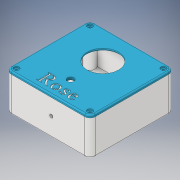
# Autodesk Inventor part: Box
Saved by Autodesk Inventor 2018.3 (Build 223284000, 284)
## iProperties
Created: 2018-06-03
Part Number: Box
Material: Generisch
Document SubType Name: Modeling
Designer: JochenAlt
Density: 1 g/cm^3
Appearance: Vorgabe
Author: JochenAlt
Autodesk Inventor part; units mm, degrees
ref_plane "YZ Plane" through (0, 0, 0) normal (1, 0, 0) x (0, 1, 0)
ref_plane "XZ Plane" through (0, 0, 0) normal (0, 1, 0) x (-1, 0, 0)
ref_plane "XY Plane" through (0, 0, 0) normal (0, 0, 1) x (1, 0, 0)
sketch "Skizze1" plane through (0, 0, 0) normal (0, 0, 1) x (1, 0, 0)
  line L0 (57, -65) -> (-57, -65)
  line L1 (-65, -57) -> (-65, 57)
  line L2 (-57, 65) -> (57, 65)
  line L3 (65, 57) -> (65, -57)
  line L4 (65, -65) -> (-65, 65) construction
  line L5 (-65, -65) -> (65, 65) construction
  arc A0 (65, 57) -> (57, 65) centre (57, 57) ccw
  line L6 (-57, 57) -> (57, 57) construction
  line L7 (57, 57) -> (57, -57) construction
  line L8 (57, -57) -> (-57, -57) construction
  line L9 (-57, -57) -> (-57, 57) construction
  circle A1 centre (-57, 57) radius 1.5
  circle A2 centre (57, 57) radius 1.5
  circle A3 centre (-57, -57) radius 1.5
  circle A4 centre (57, -57) radius 1.5
  circle A5 centre (-57, 57) radius 4
  circle A6 centre (57, 57) radius 4
  circle A7 centre (-57, -57) radius 4
  circle A8 centre (57, -57) radius 4
  line L10 (50.755, 62) -> (-50.755, 62)
  line L11 (-62, 50.755) -> (-62, -50.755)
  line L12 (-50.755, -62) -> (50.755, -62)
  line L13 (62, -50.755) -> (62, 50.755)
  arc A9 (-65, -57) -> (-57, -65) centre (-57, -57) ccw
  arc A10 (-50.755, -62) -> (-62, -50.755) centre (-57, -57) ccw
  arc A11 (62, -50.755) -> (50.755, -62) centre (57, -57) ccw
  arc A12 (50.755, 62) -> (62, 50.755) centre (57, 57) ccw
  arc A13 (-57, 65) -> (-65, 57) centre (-57, 57) ccw
  arc A14 (-62, 50.755) -> (-50.755, 62) centre (-57, 57) ccw
  line L14 (-62, 50.755) -> (-62, 62) construction
  line L15 (-50.755, 62) -> (-62, 62) construction
  line L16 (50.755, 62) -> (62, 62) construction
  line L17 (62, 50.755) -> (62, 62) construction
  line L18 (-62, -50.755) -> (-62, -62) construction
  line L19 (-50.755, -62) -> (-62, -62) construction
  line L20 (50.755, -62) -> (62, -62) construction
  line L21 (62, -50.755) -> (62, -62) construction
  line L22 (-55.1236, 60.25) -> (-53.2472, 57)
  line L23 (-53.2472, 57) -> (-55.1236, 53.75)
  line L24 (-55.1236, 53.75) -> (-58.8764, 53.75)
  line L25 (-58.8764, 53.75) -> (-60.7528, 57)
  line L26 (-60.7528, 57) -> (-58.8764, 60.25)
  line L27 (-58.8764, 60.25) -> (-55.1236, 60.25)
  line L28 (58.8764, 60.25) -> (60.7528, 57)
  line L29 (60.7528, 57) -> (58.8764, 53.75)
  line L30 (58.8764, 53.75) -> (55.1236, 53.75)
  line L31 (55.1236, 53.75) -> (53.2472, 57)
  line L32 (53.2472, 57) -> (55.1236, 60.25)
  line L33 (55.1236, 60.25) -> (58.8764, 60.25)
  line L34 (55.1236, -53.75) -> (58.8764, -53.75)
  line L35 (58.8764, -53.75) -> (60.7528, -57)
  line L36 (60.7528, -57) -> (58.8764, -60.25)
  line L37 (58.8764, -60.25) -> (55.1236, -60.25)
  line L38 (55.1236, -60.25) -> (53.2472, -57)
  line L39 (53.2472, -57) -> (55.1236, -53.75)
  line L40 (-53.2472, -57) -> (-55.1236, -60.25)
  line L41 (-55.1236, -60.25) -> (-58.8764, -60.25)
  line L42 (-58.8764, -60.25) -> (-60.7528, -57)
  line L43 (-60.7528, -57) -> (-58.8764, -53.75)
  line L44 (-58.8764, -53.75) -> (-55.1236, -53.75)
  line L45 (-55.1236, -53.75) -> (-53.2472, -57)
  arc A15 (57, -65) -> (65, -57) centre (57, -57) ccw
  point P0 (0, 0)
  dimension "d0" = 130
  dimension "d1" = 130
  dimension "d3" = 3
  dimension "d4" = 8
  dimension "d11" = 8
  dimension "d12" = 3
  dimension "d54" = 6.5
  constraints: 92 end point, 16 centre point, 16 point on circle, 15 point on line, 14 coincident, 12 equal radius, 11 perpendicular, 6 parallel, 6 tangent, 5 equal length, 4 horizontal, 2 midpoint, 2 vertical, 1 collinear, 52 other
  measures "d0" distance of L4.end L5.end
  measures "d1" distance of L5.end L4.start
  measures "d3" diameter of A1
  measures "d4" diameter of A5
  measures "d11" radius of A13
  measures "d12" distance between parallel lines of L10 L2
  measures "d54" distance between parallel lines of L24 L27
extrude "Extrusion1" add sketch "Skizze1" along normal blind 2 contours L0 A9 L1 A13 L2 A0 L3 A15 | A12 L13 A11 L12 A10 L11 A14 L10
extrude "Extrusion2" add sketch "Skizze1" along normal blind 2 from surface at 2 contours L0 A9 L1 A13 L2 A0 L3 A15 | A5 | A6 | A7 | A8 | A12 L13 A11 L12 A10 L11 A14 L10 | L22 L23 L24 L25 L26 L27 | L28 L29 L30 L31 L32 L33 | L34 L35 L36 L37 L38 L39 | L40 L41 L42 L43 L44 L45
extrude "Extrusion3" add sketch "Skizze1" along normal blind 50 from surface at 4 contours L0 A9 L1 A13 L2 A0 L3 A15 | A5 | A6 | A7 | A8 | L22 L23 L24 L25 L26 L27 | L28 L29 L30 L31 L32 L33 | L34 L35 L36 L37 L38 L39 | L40 L41 L42 L43 L44 L45
extrude "Extrusion4" add sketch "Skizze1" along normal blind 2 from surface at 54 separate body contours L0 A9 L1 A13 L2 A0 L3 A15 | A5 | A6 | A7 | A8 | A12 L13 A11 L12 A10 L11 A14 L10 | L22 L23 L24 L25 L26 L27 | L28 L29 L30 L31 L32 L33 | L34 L35 L36 L37 L38 L39 | L40 L41 L42 L43 L44 L45
extrude "Extrusion5" add sketch "Skizze1" along normal blind 2 from surface at 56 contours L0 A9 L1 A13 L2 A0 L3 A15 | A12 L13 A11 L12 A10 L11 A14 L10 bodies 2
extrude "Extrusion9" cut sketch "Skizze1" against normal blind 12 from surface at 54 contours L22 L23 L24 L25 L26 L27 | L28 L29 L30 L31 L32 L33 | L34 L35 L36 L37 L38 L39 | L40 L41 L42 L43 L44 L45 bodies 1
fillet "Rundung1" radius 2 7 edges at (65, 0, 0) (62.6569, 62.6569, 0) (0, 65, 0) (-62.6569, 62.6569, 0) (-65, 0, 0) (-62.6569, -62.6569, 0) (0, -65, 0)
fillet "Rundung2" radius 2 7 edges at (-62.6569, -62.6569, 58) (-65, 0, 58) (-62.6569, 62.6569, 58) (0, 65, 58) (62.6569, 62.6569, 58) (65, 0, 58) (0, -65, 58)
sketch "Skizze2" plane through (-57, 63, 58) normal (0, 0, 1) x (1, 0, 0)
  circle A0 centre (57, -43) radius 24.25
  circle A1 centre (57, -43) radius 25.5
  circle A2 centre (57, -93) radius 5
  circle A3 centre (57, -43) radius 28.5
  circle A4 centre (57, -43) radius 29
  point P0 (57, -63)
  dimension "d22" = 48.5
  dimension "d28" = 51
  dimension "d29" = 20
  dimension "d30" = 10
  dimension "d31" = 50
  dimension "d63" = 3
  dimension "d68" = 0.5
  constraints: 5 centre point, 3 coincident
  measures "d22" diameter of A0
  measures "d28" diameter of A1
  measures "d29" distance of A0.centre point (57, -63)
  measures "d30" diameter of A2
  measures "d31" distance of A2.centre A0.centre
  measures "d63" radial gap between concentric circles of A3 A1
  measures "d68" radial gap between concentric circles of A4 A3
extrude "Extrusion6" cut sketch "Skizze2" against normal up to next contours A0 | A2 bodies 2
extrude "Extrusion7" cut sketch "Skizze2" along normal blind 2 from surface at -4 contours A1 bodies 2
sketch "Odroid" plane through (0, 0, 0) normal (0, 0, 1) x (1, 0, 0)
  line L0 (-51, 9.5) -> (7, 9.5) construction
  line L1 (7, 9.5) -> (7, -39.5) construction
  line L2 (7, -39.5) -> (-51, -39.5) construction
  line L3 (-51, -39.5) -> (-51, 9.5) construction
  circle A0 centre (-51, 9.5) radius 1.4
  circle A1 centre (7, 9.5) radius 1.4
  circle A2 centre (7, -39.5) radius 1.4
  circle A3 centre (-51, -39.5) radius 1.4
  line L4 (-52.5, 13) -> (28.5, 13)
  line L5 (30.5, 11) -> (30.5, -41)
  line L6 (28.5, -43) -> (-52.5, -43)
  line L7 (-54.5, -41) -> (-54.5, 11)
  line L8 (-54.5, 13) -> (30.5, -43) construction
  line L9 (-54.5, -43) -> (30.5, 13) construction
  line L10 (-51, -15) -> (7, -15) construction
  arc A4 (-52.5, 13) -> (-54.5, 11) centre (-52.5, 11) ccw
  arc A5 (30.5, 11) -> (28.5, 13) centre (28.5, 11) ccw
  arc A6 (28.5, -43) -> (30.5, -41) centre (28.5, -41) ccw
  arc A7 (-54.5, -41) -> (-52.5, -43) centre (-52.5, -41) ccw
  circle A8 centre (-51, -39.5) radius 2.5
  circle A9 centre (7, -39.5) radius 2.5
  circle A10 centre (7, 9.5) radius 2.5
  circle A11 centre (-51, 9.5) radius 2.5
  line L11 (-54.5, 42) -> (-0.5, 42)
  line L12 (-0.5, 42) -> (-0.5, 18)
  line L13 (-0.5, 18) -> (-54.5, 18)
  line L14 (-54.5, 18) -> (-54.5, 42)
  circle A12 centre (-45.7, 39.5) radius 2.5
  circle A13 centre (-9.3, 20.5) radius 2.5
  circle A14 centre (-9.3, 20.5) radius 1.4
  circle A15 centre (-45.7, 39.5) radius 1.4
  line L15 (0.5, 42) -> (54.5, 42)
  line L16 (54.5, 42) -> (54.5, 18)
  line L17 (54.5, 18) -> (0.5, 18)
  line L18 (0.5, 18) -> (0.5, 42)
  circle A16 centre (9.3, 39.5) radius 2.5
  circle A17 centre (45.7, 20.5) radius 2.5
  circle A18 centre (45.7, 20.5) radius 1.4
  circle A19 centre (9.3, 39.5) radius 1.4
  line L19 (50.755, 62) -> (-50.755, 62) construction
  arc A20 (-62, 50.755) -> (-50.755, 62) centre (-57, 57) ccw construction
  line L20 (-62, 50.755) -> (-62, -50.755) construction
  arc A21 (-50.755, -62) -> (-62, -50.755) centre (-57, -57) ccw construction
  line L21 (-50.755, -62) -> (50.755, -62) construction
  arc A22 (62, -50.755) -> (50.755, -62) centre (57, -57) ccw construction
  line L22 (62, -50.755) -> (62, 50.755) construction
  arc A23 (50.755, 62) -> (62, 50.755) centre (57, 57) ccw construction
  line L23 (0, 91) -> (0, -91) construction
  line L24 (-91, 0) -> (91, 0) construction
  point P0 (0, 0)
  point P1 (-12, -15)
  point P2 (-12, -15)
  dimension "d32" = 58
  dimension "d33" = 49
  dimension "d34" = 2.8
  dimension "d35" = 56
  dimension "d36" = 85
  dimension "d37" = 3.5
  dimension "d38" = 15
  dimension "d39" = 12
  dimension "d40" = 2
  dimension "d41" = 5
  dimension "d47" = 24
  dimension "d49" = 2.5
  dimension "d50" = 2.5
  dimension "d51" = 8.8
  dimension "d53" = 8.8
  dimension "d73" = 24
  dimension "d74" = 2.5
  dimension "d75" = 2.5
  dimension "d76" = 8.8
  dimension "d77" = 8.8
  dimension "d78" = 1
  dimension "d87" = 54
  dimension "d88" = 20
  constraints: 38 end point, 20 centre point, 15 equal radius, 12 coincident, 9 point on line, 8 parallel, 8 point on circle, 8 tangent, 4 horizontal, 4 midpoint, 4 perpendicular, 2 collinear, 1 other
  measures "d32" distance of L0.start L0.end
  measures "d33" distance of L0.end L1.end
  measures "d34" diameter of A0
  measures "d35" distance of L9.end L8.end
  measures "d36" distance of L8.start L9.end
  measures "d37" distance between parallel lines of L3 L7
  measures "d38" vertical distance of point (-12, -15) point (0, 0)
  measures "d39" horizontal distance of point (-12, -15) point (0, 0)
  measures "d40" radius of A4
  measures "d41" diameter of A8
  measures "d47" distance of L11.end L12.end
  measures "d49" distance from line of L11 A12.centre
  measures "d50" distance from line of L13 A13.centre
  measures "d51" distance from line of A12.centre L14
  measures "d53" distance from line of L12 A13.centre
  measures "d73" distance of L16.start L16.end
  measures "d74" distance from line of L15 A16.centre
  measures "d75" distance from line of L17 A17.centre
  measures "d76" distance from line of A16.centre L18
  measures "d77" distance from line of L16 A17.centre
  measures "d78" distance between parallel lines of L18 L12
  measures "d87" distance of L11.start L11.end
  measures "d88" distance between parallel lines of L15 L19
extrude "Extrusion8" add sketch "Odroid" along normal blind 5 from surface at 4 contours A8 | A9 | A10 | A11 | A13 | A12 | A17 | A16 bodies 1
sketch "Skizze5" plane through (-57, -65, 54) normal (0, -1, 0) x (1, 0, 0)
  line L0 (0, -52) -> (0, 0) construction
  line L1 (114, -52) -> (0, -52) construction
  line L2 (114, 0) -> (0, 0) construction
  circle A0 centre (62, -25) radius 2.5
  line L3 (114, -52) -> (114, 0) projected
  point P0 (57, -54)
  dimension "d59" = 5
  dimension "d60" = 25
  constraints: 1 centre point
  measures "d59" diameter of A0
  measures "d60" distance from line of A0.centre L2
extrude "Extrusion10" cut sketch "Skizze5" against normal up to surface (3 mm away) bodies 1
extrude "Extrusion11" add sketch "Skizze2" against normal blind 2 from surface at -4 separate body contours A1 | A3
extrude "Extrusion12" cut sketch "Skizze2" along normal blind 0.5 from surface at -4 contours A0 | A1 | A3 | A4 bodies 2
sketch "Skizze6" plane through (-57, -63, 58) normal (0, 0, 1) x (1, 0, 0)
  line L0 (50.0673, 25.5729) -> (65.8585, 25.5729) construction
  line L1 (65.8585, 25.5729) -> (65.8585, 18.3705) construction
  line L2 (65.8585, 18.3705) -> (50.0673, 18.3705) construction
  line L3 (50.0673, 18.3705) -> (50.0673, 25.5729) construction
  circle A0 centre (57, 33) radius 5 construction
  circle A1 centre (114, 6) radius 4 construction
  circle A2 centre (0, 6) radius 4 construction
  circle A3 centre (114, 120) radius 4 construction
  circle A4 centre (0, 120) radius 4 construction
  arc A5 (-6, 6) -> (0, 0) centre (0, 6) ccw construction
  line L4 (114, 0) -> (0, 0) construction
  line L5 (120, 120) -> (120, 6) construction
  arc A6 (120, 120) -> (114, 126) centre (114, 120) ccw construction
  line L6 (0, 126) -> (114, 126) construction
  arc A7 (0, 126) -> (-6, 120) centre (0, 120) ccw construction
  line L7 (-6, 6) -> (-6, 120) construction
  circle A8 centre (57, 83) radius 24.25 construction
  circle A9 centre (57, 83) radius 29 construction
  circle A10 centre (57, 33) radius 5 construction
  circle A11 centre (0, 120) radius 1.5 construction
  circle A12 centre (114, 120) radius 1.5 construction
  circle A13 centre (0, 6) radius 1.5 construction
  circle A14 centre (114, 6) radius 1.5 construction
  arc A15 (0, 128) -> (-8, 120) centre (0, 120) ccw construction
  line L8 (0, 128) -> (114, 128) construction
  arc A16 (122, 120) -> (114, 128) centre (114, 120) ccw construction
  line L9 (122, 120) -> (122, 6) construction
  line L10 (114, -2) -> (0, -2) construction
  arc A17 (-8, 6) -> (0, -2) centre (0, 6) ccw construction
  line L11 (-8, 6) -> (-8, 120) construction
  arc A18 (114, 0) -> (120, 6) centre (114, 6) ccw projected
  arc A19 (114, -2) -> (122, 6) centre (114, 6) ccw projected
  spline S0 degree 2 poles (47.4778, 6.3729) (47.4948, 6.0325) (46.9161, 6.0325) knots 0 0 0 1 1 1
  spline S1 degree 2 poles (46.9161, 6.0325) (41.6565, 6.0325) (36.9927, 15.0197) knots 0 0 0 1 1 1
  spline S2 degree 2 poles (36.9927, 15.0197) (35.1884, 14.9346) (35.0693, 14.9346) knots 0 0 0 1 1 1
  line L12 (35.0693, 14.9346) -> (35.0693, 8.7899)
  spline S3 degree 2 poles (35.0693, 8.7899) (35.0693, 8.1091) (35.7501, 7.6495) (36.9076, 7.4793) knots 0 0 0 1 2 2 2
  spline S4 degree 2 poles (36.9076, 7.4793) (37.7076, 7.3431) (37.7076, 6.9006) knots 0 0 0 1 1 1
  spline S5 degree 2 poles (37.7076, 6.9006) (37.7076, 6.5431) (37.4522, 6.3729) (36.8395, 6.407) knots 0 0 0 1 2 2 2
  spline S6 degree 2 poles (36.8395, 6.407) (34.2012, 6.5261) (31.0693, 6.2878) knots 0 0 0 1 1 1
  spline S7 degree 2 poles (31.0693, 6.2878) (30.4395, 6.2368) (30.4395, 6.7985) knots 0 0 0 1 1 1
  spline S8 degree 2 poles (30.4395, 6.7985) (30.4395, 7.1729) (31.0693, 7.224) knots 0 0 0 1 1 1
  spline S9 degree 2 poles (31.0693, 7.224) (32.499, 7.3772) (32.499, 8.7899) knots 0 0 0 1 1 1
  line L13 (32.499, 8.7899) -> (32.499, 22.7985)
  spline S10 degree 2 poles (32.499, 22.7985) (32.499, 24.1942) (30.865, 24.5176) knots 0 0 0 1 1 1
  spline S11 degree 2 poles (30.865, 24.5176) (30.065, 24.6708) (30.065, 25.0282) knots 0 0 0 1 1 1
  spline S12 degree 2 poles (30.065, 25.0282) (30.065, 25.5729) (30.6097, 25.5729) knots 0 0 0 1 1 1
  spline S13 degree 2 poles (30.6097, 25.5729) (30.7629, 25.5729) (30.9501, 25.5389) knots 0 0 0 1 1 1
  spline S14 degree 2 poles (30.9501, 25.5389) (31.5629, 25.4538) (32.7884, 25.4538) knots 0 0 0 1 1 1
  spline S15 degree 2 poles (32.7884, 25.4538) (33.1969, 25.4538) (36.499, 25.5389) (37.9288, 25.5389) knots 0 0 0 1 2 2 2
  spline S16 degree 2 poles (37.9288, 25.5389) (40.8565, 25.5389) (42.5416, 24.4495) knots 0 0 0 1 1 1
  spline S17 degree 2 poles (42.5416, 24.4495) (44.448, 23.224) (44.448, 20.858) knots 0 0 0 1 1 1
  spline S18 degree 2 poles (44.448, 20.858) (44.448, 16.807) (39.7671, 15.5134) knots 0 0 0 1 1 1
  spline S19 degree 2 poles (39.7671, 15.5134) (41.265, 12.1091) (43.2735, 9.6921) knots 0 0 0 1 1 1
  spline S20 degree 2 poles (43.2735, 9.6921) (45.3501, 7.1899) (47.0012, 6.9346) knots 0 0 0 1 1 1
  spline S21 degree 2 poles (47.0012, 6.9346) (47.4437, 6.8665) (47.4778, 6.3729) knots 0 0 0 1 1 1
  spline S22 degree 2 poles (41.5884, 20.5006) (41.5884, 22.6793) (39.3586, 24.5176) (36.9246, 24.5176) knots 0 0 0 1 2 2 2
  spline S23 degree 2 poles (36.9246, 24.5176) (35.8352, 24.5176) (35.0693, 23.9219) (35.0693, 22.9176) knots 0 0 0 1 2 2 2
  line L14 (35.0693, 22.9176) -> (35.0693, 16.024)
  spline S24 degree 2 poles (35.0693, 16.024) (38.6097, 16.1431) (40.1586, 17.2665) knots 0 0 0 1 1 1
  spline S25 degree 2 poles (40.1586, 17.2665) (41.5884, 18.3048) (41.5884, 20.5006) knots 0 0 0 1 1 1
  spline S26 degree 2 poles (61.6054, 12.2963) (61.6054, 9.7431) (57.8267, 6.2197) (55.0352, 6.2197) knots 0 0 0 1 2 2 2
  spline S27 degree 2 poles (55.0352, 6.2197) (52.2437, 6.2197) (50.6267, 7.7687) knots 0 0 0 1 1 1
  spline S28 degree 2 poles (50.6267, 7.7687) (49.0608, 9.2836) (49.0608, 11.7857) knots 0 0 0 1 1 1
  spline S29 degree 2 poles (49.0608, 11.7857) (49.0608, 14.3729) (51.0352, 16.1431) knots 0 0 0 1 1 1
  spline S30 degree 2 poles (51.0352, 16.1431) (52.9416, 17.8623) (55.6139, 17.8623) knots 0 0 0 1 1 1
  spline S31 degree 2 poles (55.6139, 17.8623) (58.4565, 17.8623) (60.0565, 16.3304) knots 0 0 0 1 1 1
  spline S32 degree 2 poles (60.0565, 16.3304) (61.6054, 14.8325) (61.6054, 12.2963) knots 0 0 0 1 1 1
  spline S33 degree 2 poles (59.0352, 11.3942) (59.0352, 13.6921) (57.9288, 15.1219) knots 0 0 0 1 1 1
  spline S34 degree 2 poles (57.9288, 15.1219) (56.8395, 16.5176) (55.1714, 16.5176) knots 0 0 0 1 1 1
  spline S35 degree 2 poles (55.1714, 16.5176) (53.6225, 16.5176) (51.665, 14.3389) (51.665, 12.7729) knots 0 0 0 1 2 2 2
  spline S36 degree 2 poles (51.665, 12.7729) (51.665, 10.2538) (52.8054, 8.858) knots 0 0 0 1 1 1
  spline S37 degree 2 poles (52.8054, 8.858) (53.8608, 7.5644) (55.5629, 7.5644) knots 0 0 0 1 1 1
  spline S38 degree 2 poles (55.5629, 7.5644) (57.1629, 7.5644) (59.0352, 9.6921) (59.0352, 11.3942) knots 0 0 0 1 2 2 2
  spline S39 degree 2 poles (73.1288, 9.5389) (73.1288, 7.9899) (70.7459, 6.1517) (68.6863, 6.1517) knots 0 0 0 1 2 2 2
  spline S40 degree 2 poles (68.6863, 6.1517) (67.3076, 6.1517) (65.9288, 6.441) knots 0 0 0 1 1 1
  spline S41 degree 2 poles (65.9288, 6.441) (64.7373, 6.7134) (64.5501, 6.9346) knots 0 0 0 1 1 1
  spline S42 degree 2 poles (64.5501, 6.9346) (64.431, 7.1389) (64.431, 8.9261) knots 0 0 0 1 1 1
  spline S43 degree 2 poles (64.431, 8.9261) (64.431, 9.6921) (64.7884, 9.7261) knots 0 0 0 1 1 1
  spline S44 degree 2 poles (64.7884, 9.7261) (65.1288, 9.7772) (65.3842, 9.3517) knots 0 0 0 1 1 1
  spline S45 degree 2 poles (65.3842, 9.3517) (66.4905, 7.4453) (68.9416, 7.4453) knots 0 0 0 1 1 1
  spline S46 degree 2 poles (68.9416, 7.4453) (71.0012, 7.4453) (71.0012, 8.8751) knots 0 0 0 1 1 1
  spline S47 degree 2 poles (71.0012, 8.8751) (71.0012, 9.5048) (70.5246, 9.9304) knots 0 0 0 1 1 1
  spline S48 degree 2 poles (70.5246, 9.9304) (70.0139, 10.407) (68.5331, 11.0538) knots 0 0 0 1 1 1
  spline S49 degree 2 poles (68.5331, 11.0538) (66.4054, 12.007) (65.6905, 12.7219) knots 0 0 0 1 1 1
  spline S50 degree 2 poles (65.6905, 12.7219) (64.9076, 13.4878) (64.9076, 14.7814) knots 0 0 0 1 1 1
  spline S51 degree 2 poles (64.9076, 14.7814) (64.9076, 16.3644) (66.1161, 17.2325) knots 0 0 0 1 1 1
  spline S52 degree 2 poles (66.1161, 17.2325) (67.2565, 18.0836) (69.1288, 18.0836) knots 0 0 0 1 1 1
  spline S53 degree 2 poles (69.1288, 18.0836) (70.3203, 18.0836) (71.3076, 17.8963) knots 0 0 0 1 1 1
  spline S54 degree 2 poles (71.3076, 17.8963) (72.3459, 17.6921) (72.3969, 17.4197) knots 0 0 0 1 1 1
  spline S55 degree 2 poles (72.3969, 17.4197) (72.5161, 16.6027) (72.8735, 15.0538) knots 0 0 0 1 1 1
  spline S56 degree 2 poles (72.8735, 15.0538) (72.9246, 14.8665) (72.465, 14.7474) knots 0 0 0 1 1 1
  spline S57 degree 2 poles (72.465, 14.7474) (71.9714, 14.6453) (71.8182, 14.9006) knots 0 0 0 1 1 1
  spline S58 degree 2 poles (71.8182, 14.9006) (70.6608, 16.7899) (68.8905, 16.7899) knots 0 0 0 1 1 1
  spline S59 degree 2 poles (68.8905, 16.7899) (66.899, 16.7899) (66.899, 15.5134) knots 0 0 0 1 1 1
  spline S60 degree 2 poles (66.899, 15.5134) (66.899, 14.7814) (67.4437, 14.3729) knots 0 0 0 1 1 1
  spline S61 degree 2 poles (67.4437, 14.3729) (67.9203, 13.9985) (69.7076, 13.2155) knots 0 0 0 1 1 1
  spline S62 degree 2 poles (69.7076, 13.2155) (71.5799, 12.4155) (72.2437, 11.7687) knots 0 0 0 1 1 1
  spline S63 degree 2 poles (72.2437, 11.7687) (73.1288, 10.9346) (73.1288, 9.5389) knots 0 0 0 1 1 1
  spline S64 degree 2 poles (86.7459, 8.841) (86.7459, 8.2112) (85.0437, 7.2751) knots 0 0 0 1 1 1
  spline S65 degree 2 poles (85.0437, 7.2751) (83.1203, 6.2368) (81.0778, 6.2368) knots 0 0 0 1 1 1
  spline S66 degree 2 poles (81.0778, 6.2368) (78.865, 6.2368) (77.3671, 7.6836) knots 0 0 0 1 1 1
  spline S67 degree 2 poles (77.3671, 7.6836) (75.7501, 9.2325) (75.7501, 11.7857) knots 0 0 0 1 1 1
  spline S68 degree 2 poles (75.7501, 11.7857) (75.7501, 14.6793) (77.5544, 16.4495) knots 0 0 0 1 1 1
  spline S69 degree 2 poles (77.5544, 16.4495) (79.2395, 18.0836) (81.6735, 18.0836) knots 0 0 0 1 1 1
  spline S70 degree 2 poles (81.6735, 18.0836) (83.1203, 18.0836) (84.3799, 17.1644) knots 0 0 0 1 1 1
  spline S71 degree 2 poles (84.3799, 17.1644) (85.5203, 16.3304) (85.8778, 15.2751) knots 0 0 0 1 1 1
  spline S72 degree 2 poles (85.8778, 15.2751) (86.0139, 14.9176) (86.2693, 14.8665) knots 0 0 0 1 1 1
  spline S73 degree 2 poles (86.2693, 14.8665) (86.6608, 14.7985) (86.6608, 14.3559) knots 0 0 0 1 1 1
  spline S74 degree 2 poles (86.6608, 14.3559) (86.6608, 13.7431) (85.2139, 13.3176) knots 0 0 0 1 1 1
  line L15 (85.2139, 13.3176) -> (78.4735, 11.3261)
  spline S75 degree 2 poles (78.4735, 11.3261) (79.1373, 7.8538) (82.048, 7.8538) knots 0 0 0 1 1 1
  spline S76 degree 2 poles (82.048, 7.8538) (83.7331, 7.8538) (85.8778, 9.0793) knots 0 0 0 1 1 1
  spline S77 degree 2 poles (85.8778, 9.0793) (86.2012, 9.2665) (86.5246, 9.2665) knots 0 0 0 1 1 1
  spline S78 degree 2 poles (86.5246, 9.2665) (86.7459, 9.2665) (86.7459, 8.841) knots 0 0 0 1 1 1
  spline S79 degree 2 poles (83.2735, 14.7134) (83.2735, 15.5134) (81.9629, 16.7389) (81.0097, 16.7389) knots 0 0 0 1 2 2 2
  spline S80 degree 2 poles (81.0097, 16.7389) (78.3203, 16.7389) (78.3203, 12.841) knots 0 0 0 1 1 1
  line L16 (78.3203, 12.841) -> (78.3203, 12.5006)
  line L17 (78.3203, 12.5006) -> (82.3033, 13.6921)
  spline S81 degree 2 poles (82.3033, 13.6921) (83.2735, 13.9644) (83.2735, 14.7134) knots 0 0 0 1 1 1
  point P0 (57, 63)
  constraints: 1 coincident, 2 other
extrude "Extrusion13" cut sketch "Skizze6" against normal blind 1 bodies 2
sketch "Skizze7" plane through (-57, 65, 54) normal (0, 1, 0) x (1, 0, 0)
  line L0 (114, 52) -> (114, 0) construction
  line L1 (0, 52) -> (114, 52) construction
  line L2 (0, 0) -> (0, 52) construction
  line L3 (0, 0) -> (114, 0) construction
  circle A0 centre (57, 30) radius 5
  line L4 (0, 52) -> (114, 52) construction
  line L5 (57, 52) -> (57, 0) construction
  line L6 (0, 0) -> (114, 0) construction
  circle A1 centre (57, 15) radius 3.5
  point P0 (57, 54)
  dimension "d80" = 10
  dimension "d81" = 30
  dimension "d83" = 7
  dimension "d84" = 15
  constraints: 2 centre point, 2 end point, 2 midpoint, 2 point on line
  measures "d80" diameter of A0
  measures "d81" distance from line of A0.centre L3
  measures "d83" diameter of A1
  measures "d84" distance of A1.centre A0.centre
extrude "Extrusion14" cut sketch "Skizze7" against normal up to surface (3 mm away) bodies 1
equation "\"d50\" = d49"
equation "\"d75\" = d74"
